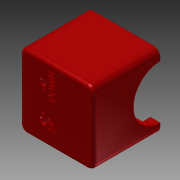
# Autodesk Inventor part: Durometer_Electronics_Enclosure_Lid
Saved by Autodesk Inventor 2015 (Build 190159000, 159)
## iProperties
Created: 2015-01-04
Part Number: Durometer_Electronics_Enclosure_Lid
Material: Generic
Document SubType Name: Modeling
Designer: Drew
Density: 1 g/cm^3
Appearance: Smooth - Red
Author: Drew
Autodesk Inventor part; units mm, degrees
ref_plane "YZ Plane" through (0, 0, 0) normal (1, 0, 0) x (0, 1, 0)
ref_plane "XZ Plane" through (0, 0, 0) normal (0, 1, 0) x (-1, 0, 0)
ref_plane "XY Plane" through (0, 0, 0) normal (0, 0, 1) x (1, 0, 0)
sketch "Sketch1" plane through (0, 0, 0) normal (0, 0, 1) x (1, 0, 0)
  line L0 (28.575, -34.925) -> (-28.575, -34.925)
  line L1 (-34.925, -28.575) -> (-34.925, 28.575)
  line L2 (-28.575, 34.925) -> (28.575, 34.925)
  line L3 (34.925, 28.575) -> (34.925, -28.575)
  line L4 (34.925, -34.925) -> (-34.925, 34.925) construction
  line L5 (-34.925, -34.925) -> (34.925, 34.925) construction
  arc A0 (-28.575, 34.925) -> (-34.925, 28.575) centre (-28.575, 28.575) ccw
  arc A1 (34.925, 28.575) -> (28.575, 34.925) centre (28.575, 28.575) ccw
  arc A2 (28.575, -34.925) -> (34.925, -28.575) centre (28.575, -28.575) ccw
  arc A3 (-34.925, -28.575) -> (-28.575, -34.925) centre (-28.575, -28.575) ccw
  point P0 (0, 0)
  dimension "d0" = 69.85
  dimension "d1" = 69.85
  dimension "d2" = 6.35
  constraints: 12 end point, 8 point on circle, 8 point on line, 8 tangent, 4 centre point, 3 equal radius, 2 midpoint, 2 parallel, 1 horizontal, 1 perpendicular
  measures "d0" distance of L4.end L5.end
  measures "d1" distance between parallel lines of L0 L2
  measures "d2" radius of A0
extrude "Extrusion1" add sketch "Sketch1" along normal blind 63.5
shell "Shell1" thickness 2.032 removed faces 1 at (9.525, 7.4083, 0)
sketch "Sketch4" plane through (0, 0, 0) normal (0, 0, -1) x (-1, 0, 0)
  arc A0 (-32.893, -28.575) -> (-28.575, -32.893) centre (-28.575, -28.575) ccw projected
  line L0 (-43.2886, 0) -> (36.2185, 0)
  line L1 (0, 45.1294) -> (0, -40.5019)
  line L2 (-28.575, -24.257) -> (-32.893, -24.257)
  line L3 (-24.257, -28.575) -> (-24.257, -32.893)
  line L4 (-24.257, -32.893) -> (-28.575, -32.893)
  line L5 (-32.893, -24.257) -> (-32.893, -28.575)
  arc A1 (-32.893, -28.575) -> (-28.575, -32.893) centre (-28.575, -28.575) ccw
  arc A2 (-24.257, -28.575) -> (-28.575, -24.257) centre (-28.575, -28.575) ccw
  arc A3 (-28.575, 32.893) -> (-32.893, 28.575) centre (-28.575, 28.575) ccw
  line L6 (-28.575, 24.257) -> (-32.893, 24.257)
  line L7 (-24.257, 28.575) -> (-24.257, 32.893)
  line L8 (-24.257, 32.893) -> (-28.575, 32.893)
  line L9 (-32.893, 24.257) -> (-32.893, 28.575)
  arc A4 (-28.575, 32.893) -> (-32.893, 28.575) centre (-28.575, 28.575) ccw
  arc A5 (-28.575, 24.257) -> (-24.257, 28.575) centre (-28.575, 28.575) ccw
  arc A6 (28.575, -32.893) -> (32.893, -28.575) centre (28.575, -28.575) ccw
  line L10 (28.575, -24.257) -> (32.893, -24.257)
  line L11 (24.257, -28.575) -> (24.257, -32.893)
  line L12 (24.257, -32.893) -> (28.575, -32.893)
  line L13 (32.893, -24.257) -> (32.893, -28.575)
  arc A7 (28.575, -32.893) -> (32.893, -28.575) centre (28.575, -28.575) ccw
  arc A8 (28.575, -24.257) -> (24.257, -28.575) centre (28.575, -28.575) ccw
  arc A9 (32.893, 28.575) -> (28.575, 32.893) centre (28.575, 28.575) ccw
  line L14 (28.575, 24.257) -> (32.893, 24.257)
  line L15 (24.257, 28.575) -> (24.257, 32.893)
  line L16 (24.257, 32.893) -> (28.575, 32.893)
  line L17 (32.893, 24.257) -> (32.893, 28.575)
  arc A10 (32.893, 28.575) -> (28.575, 32.893) centre (28.575, 28.575) ccw
  arc A11 (24.257, 28.575) -> (28.575, 24.257) centre (28.575, 28.575) ccw
  circle A12 centre (-28.575, -28.575) radius 1.45
  circle A13 centre (-28.575, 28.575) radius 1.45
  circle A14 centre (28.575, -28.575) radius 1.45
  circle A15 centre (28.575, 28.575) radius 1.45
  point P0 (0, 0)
  dimension "d7" = 4.318
  dimension "d8" = 4.318
  dimension "d11" = 2.9
  constraints: 36 end point, 27 symmetric about line, 22 point on circle, 15 centre point, 5 coincident, 4 tangent, 2 horizontal, 2 point on line, 1 vertical, 12 other
  measures "d7" distance of L2.end L5.end
  measures "d8" distance of L3.start L3.end
  measures "d11" diameter of A12
extrude "Extrusion2" add sketch "Sketch4" against normal up to surface (61.468 mm away)
fillet "Fillet2" radius 3.175 24 edges at (33.0651, 33.0651, 63.5) (0, 34.925, 63.5) (-33.0651, 33.0651, 63.5) (-34.925, 0, 63.5) (-33.0651, -33.0651, 63.5) (0, -34.925, 63.5) (33.0651, -33.0651, 63.5) (34.925, 0, 63.5) (32.893, 0, 61.468) (24.257, -30.734, 61.468) (30.734, -24.257, 61.468) (25.5217, -25.5217, 61.468) (0, -32.893, 61.468) (0, 32.893, 61.468) (30.734, 24.257, 61.468) (24.257, 30.734, 61.468) (25.5217, 25.5217, 61.468) (-30.734, -24.257, 61.468) (-24.257, -30.734, 61.468) (-25.5217, -25.5217, 61.468) (-32.893, 0, 61.468) (-24.257, 30.734, 61.468) (-30.734, 24.257, 61.468) (-25.5217, 25.5217, 61.468)
sketch "Sketch5" plane through (0, 0, 63.5) normal (0, 0, 1) x (1, 0, 0)
  circle A0 centre (-12.7, -15.875) radius 3.429
  line L0 (-50.1018, 0) -> (45.2159, 0)
  line L1 (-12.7, -24.1987) -> (-12.7, -7.4873)
  line L2 (-11.43, -9.144) -> (-13.97, -9.144)
  line L3 (-13.97, -9.144) -> (-13.97, -10.414)
  line L4 (-13.97, -10.414) -> (-11.43, -10.414)
  line L5 (-11.43, -10.414) -> (-11.43, -9.144)
  line L6 (-11.43, -9.144) -> (-13.97, -10.414) construction
  line L7 (-13.97, -9.144) -> (-11.43, -10.414) construction
  circle A1 centre (-12.7, 15.875) radius 3.429
  line L8 (-12.7, 24.1987) -> (-12.7, 7.4873)
  line L9 (-11.43, 9.144) -> (-13.97, 9.144)
  line L10 (-13.97, 9.144) -> (-13.97, 10.414)
  line L11 (-13.97, 10.414) -> (-11.43, 10.414)
  line L12 (-11.43, 10.414) -> (-11.43, 9.144)
  line L13 (-11.43, 9.144) -> (-13.97, 10.414) construction
  line L14 (-13.97, 9.144) -> (-11.43, 10.414) construction
  point P0 (0, 0)
  point P1 (-12.7, -9.779)
  point P2 (-12.7, 9.779)
  dimension "d31" = 6.096
  dimension "d32" = 6.858
  dimension "d33" = 2.54
  dimension "d34" = 1.27
  dimension "d35" = 31.75
  dimension "d36" = 12.7
  constraints: 30 end point, 8 symmetric about line, 4 midpoint, 3 point on line, 2 centre point, 2 horizontal, 2 parallel, 1 perpendicular, 1 vertical, 1 other
  measures "d31" distance of A0.centre point (-12.7, -9.779)
  measures "d32" diameter of A0
  measures "d33" distance of L2.start L2.end
  measures "d34" distance of L2.end L3.end
  measures "d35" diameter of A0.centre L0
  measures "d36" horizontal distance of point (0, 0) A0.centre
extrude "Extrusion3" cut sketch "Sketch5" against normal through all
sketch "Sketch6" plane through (0, 0, 63.5) normal (0, 0, 1) x (1, 0, 0)
  line L0 (-8.5246, -20.4603) -> (-8.5246, -15.2971) construction
  line L1 (-8.5246, -15.2971) -> (-5.3496, -15.2971) construction
  line L2 (-5.3496, -15.2971) -> (-5.3496, -20.4603) construction
  line L3 (-5.3496, -20.4603) -> (-8.5246, -20.4603) construction
  line L4 (-7.8723, 3.9052) -> (-7.8723, 16.5422) construction
  line L5 (-7.8723, 16.5422) -> (-4.6973, 16.5422) construction
  line L6 (-4.6973, 16.5422) -> (-4.6973, 3.9052) construction
  line L7 (-4.6973, 3.9052) -> (-7.8723, 3.9052) construction
  spline S0 degree 2 poles (-2.3002, -17.7136) (-2.3002, -18.2521) (-2.5818, -19.0523) (-2.8633, -19.3339) knots 0 0 0 1 2 2 2
  spline S1 degree 2 poles (-2.8633, -19.3339) (-3.1795, -19.655) (-4.0687, -19.9168) (-4.7208, -19.9168) knots 0 0 0 1 2 2 2
  line L8 (-4.7208, -19.9168) -> (-8.5246, -19.9168)
  line L9 (-8.5246, -19.9168) -> (-8.5246, -19.1067)
  line L10 (-8.5246, -19.1067) -> (-4.7208, -19.1067)
  spline S2 degree 2 poles (-4.7208, -19.1067) (-4.296, -19.1067) (-3.7229, -18.998) (-3.4907, -18.8449) knots 0 0 0 1 2 2 2
  spline S3 degree 2 poles (-3.4907, -18.8449) (-3.2437, -18.6818) (-2.9918, -18.1187) (-2.9918, -17.7136) knots 0 0 0 1 2 2 2
  spline S4 degree 2 poles (-2.9918, -17.7136) (-2.9918, -17.3332) (-3.2437, -16.7404) (-3.4907, -16.5774) knots 0 0 0 1 2 2 2
  spline S5 degree 2 poles (-3.4907, -16.5774) (-3.7229, -16.4242) (-4.291, -16.3156) (-4.701, -16.3156) knots 0 0 0 1 2 2 2
  line L11 (-4.701, -16.3156) -> (-8.5246, -16.3156)
  line L12 (-8.5246, -16.3156) -> (-8.5246, -15.5054)
  line L13 (-8.5246, -15.5054) -> (-4.7208, -15.5054)
  spline S6 degree 2 poles (-4.7208, -15.5054) (-4.0835, -15.5054) (-3.1746, -15.7623) (-2.8633, -16.0883) knots 0 0 0 1 2 2 2
  spline S7 degree 2 poles (-2.8633, -16.0883) (-2.5768, -16.3798) (-2.3002, -17.1504) (-2.3002, -17.7136) knots 0 0 0 1 2 2 2
  spline S8 degree 2 poles (-6.6869, -10.4913) (-6.2917, -10.4913) (-5.5804, -10.7728) (-5.3334, -11.0248) knots 0 0 0 1 2 2 2
  spline S9 degree 2 poles (-5.3334, -11.0248) (-5.0221, -11.341) (-4.701, -12.1956) (-4.701, -12.8477) knots 0 0 0 1 2 2 2
  line L14 (-4.701, -12.8477) -> (-4.701, -13.5343)
  line L15 (-4.701, -13.5343) -> (-2.4286, -13.5343)
  line L16 (-2.4286, -13.5343) -> (-2.4286, -14.3445)
  line L17 (-2.4286, -14.3445) -> (-8.5246, -14.3445)
  line L18 (-8.5246, -14.3445) -> (-8.5246, -12.8131)
  spline S10 degree 2 poles (-8.5246, -12.8131) (-8.5246, -12.2697) (-8.3468, -11.5089) (-8.1442, -11.2175) knots 0 0 0 1 2 2 2
  spline S11 degree 2 poles (-8.1442, -11.2175) (-7.9121, -10.8766) (-7.1957, -10.4913) (-6.6869, -10.4913) knots 0 0 0 1 2 2 2
  spline S12 degree 2 poles (-6.6622, -11.336) (-6.9784, -11.336) (-7.4428, -11.5534) (-7.591, -11.7757) knots 0 0 0 1 2 2 2
  spline S13 degree 2 poles (-7.591, -11.7757) (-7.7194, -11.9683) (-7.8231, -12.4821) (-7.8231, -12.8625) knots 0 0 0 1 2 2 2
  line L19 (-7.8231, -12.8625) -> (-7.8231, -13.5343)
  line L20 (-7.8231, -13.5343) -> (-5.3926, -13.5343)
  line L21 (-5.3926, -13.5343) -> (-5.3926, -12.981)
  spline S14 degree 2 poles (-5.3926, -12.981) (-5.3926, -12.487) (-5.5507, -11.8794) (-5.7582, -11.6818) knots 0 0 0 1 2 2 2
  spline S15 degree 2 poles (-5.7582, -11.6818) (-5.941, -11.499) (-6.3708, -11.336) (-6.6622, -11.336) knots 0 0 0 1 2 2 2
  spline S16 degree 2 poles (-4.6909, 9.3293) (-3.8561, 9.3293) (-2.5124, 8.6525) (-2.1369, 8.0844) knots 0 0 0 1 2 2 2
  spline S17 degree 2 poles (-2.1369, 8.0844) (-1.8455, 7.6201) (-1.6479, 6.6666) (-1.6479, 5.9256) knots 0 0 0 1 2 2 2
  line L22 (-1.6479, 5.9256) -> (-1.6479, 4.5227)
  line L23 (-1.6479, 4.5227) -> (-7.7439, 4.5227)
  line L24 (-7.7439, 4.5227) -> (-7.7439, 5.9108)
  spline S18 degree 2 poles (-7.7439, 5.9108) (-7.7439, 6.7704) (-7.487, 7.7485) (-7.2598, 8.0943) knots 0 0 0 1 2 2 2
  spline S19 degree 2 poles (-7.2598, 8.0943) (-6.8695, 8.6822) (-5.5802, 9.3293) (-4.6909, 9.3293) knots 0 0 0 1 2 2 2
  spline S20 degree 2 poles (-4.7008, 8.4846) (-5.4023, 8.4846) (-6.3953, 8.0202) (-6.6768, 7.5608) knots 0 0 0 1 2 2 2
  spline S21 degree 2 poles (-6.6768, 7.5608) (-6.8695, 7.2347) (-7.0424, 6.4987) (-7.0424, 5.9503) knots 0 0 0 1 2 2 2
  line L25 (-7.0424, 5.9503) -> (-7.0424, 5.3328)
  line L26 (-7.0424, 5.3328) -> (-2.3494, 5.3328)
  line L27 (-2.3494, 5.3328) -> (-2.3494, 5.9503)
  spline S22 degree 2 poles (-2.3494, 5.9503) (-2.3494, 6.4888) (-2.5223, 7.3039) (-2.7545, 7.6349) knots 0 0 0 1 2 2 2
  spline S23 degree 2 poles (-2.7545, 7.6349) (-3.041, 8.0597) (-3.9895, 8.4846) (-4.7008, 8.4846) knots 0 0 0 1 2 2 2
  spline S24 degree 2 poles (-7.0473, 14.5213) (-6.6423, 14.8671) (-5.4567, 15.2524) (-4.6959, 15.2524) knots 0 0 0 1 2 2 2
  spline S25 degree 2 poles (-4.6959, 15.2524) (-3.9549, 15.2524) (-2.7545, 14.877) (-2.3494, 14.5213) knots 0 0 0 1 2 2 2
  spline S26 degree 2 poles (-2.3494, 14.5213) (-1.9245, 14.1459) (-1.5194, 13.1529) (-1.5194, 12.5552) knots 0 0 0 1 2 2 2
  spline S27 degree 2 poles (-1.5194, 12.5552) (-1.5194, 11.9377) (-1.9393, 10.9497) (-2.3494, 10.589) knots 0 0 0 1 2 2 2
  spline S28 degree 2 poles (-2.3494, 10.589) (-2.7545, 10.2383) (-3.945, 9.8628) (-4.6959, 9.8628) knots 0 0 0 1 2 2 2
  spline S29 degree 2 poles (-4.6959, 9.8628) (-5.4616, 9.8628) (-6.6274, 10.2432) (-7.0473, 10.594) knots 0 0 0 1 2 2 2
  spline S30 degree 2 poles (-7.0473, 10.594) (-7.4524, 10.9497) (-7.8723, 11.9426) (-7.8723, 12.5552) knots 0 0 0 1 2 2 2
  spline S31 degree 2 poles (-7.8723, 12.5552) (-7.8723, 13.1776) (-7.4376, 14.1755) (-7.0473, 14.5213) knots 0 0 0 1 2 2 2
  spline S32 degree 2 poles (-4.6959, 14.4077) (-5.2986, 14.4077) (-6.2322, 14.1459) (-6.5385, 13.9087) knots 0 0 0 1 2 2 2
  spline S33 degree 2 poles (-6.5385, 13.9087) (-6.8547, 13.6667) (-7.1708, 12.9849) (-7.1708, 12.5601) knots 0 0 0 1 2 2 2
  spline S34 degree 2 poles (-7.1708, 12.5601) (-7.1708, 12.1204) (-6.8646, 11.4585) (-6.5385, 11.2065) knots 0 0 0 1 2 2 2
  spline S35 degree 2 poles (-6.5385, 11.2065) (-6.2273, 10.9645) (-5.2887, 10.7076) (-4.6959, 10.7076) knots 0 0 0 1 2 2 2
  spline S36 degree 2 poles (-4.6959, 10.7076) (-3.4955, 10.7076) (-2.2209, 11.7154) (-2.2209, 12.5601) knots 0 0 0 1 2 2 2
  spline S37 degree 2 poles (-2.2209, 12.5601) (-2.2209, 13.4048) (-3.4955, 14.4077) (-4.6959, 14.4077) knots 0 0 0 1 2 2 2
  line L28 (-7.7439, 22.9737) -> (-1.6479, 21.4423)
  line L29 (-1.6479, 21.4423) -> (-1.6479, 20.5333)
  line L30 (-1.6479, 20.5333) -> (-6.7065, 19.2934)
  line L31 (-6.7065, 19.2934) -> (-1.6479, 18.088)
  line L32 (-1.6479, 18.088) -> (-1.6479, 17.1889)
  line L33 (-1.6479, 17.1889) -> (-7.7439, 15.6328)
  line L34 (-7.7439, 15.6328) -> (-7.7439, 16.4677)
  line L35 (-7.7439, 16.4677) -> (-2.6902, 17.6928)
  line L36 (-2.6902, 17.6928) -> (-7.7439, 18.908)
  line L37 (-7.7439, 18.908) -> (-7.7439, 19.733)
  line L38 (-7.7439, 19.733) -> (-2.631, 20.9582)
  line L39 (-2.631, 20.9582) -> (-7.7439, 22.1783)
  line L40 (-7.7439, 22.1783) -> (-7.7439, 22.9737)
  line L41 (-1.6479, 28.0619) -> (-1.6479, 27.153)
  line L42 (-1.6479, 27.153) -> (-6.9041, 24.4557)
  line L43 (-6.9041, 24.4557) -> (-1.6479, 24.4557)
  line L44 (-1.6479, 24.4557) -> (-1.6479, 23.6999)
  line L45 (-1.6479, 23.6999) -> (-7.7439, 23.6999)
  line L46 (-7.7439, 23.6999) -> (-7.7439, 24.8509)
  line L47 (-7.7439, 24.8509) -> (-2.9175, 27.3061)
  line L48 (-2.9175, 27.3061) -> (-7.7439, 27.3061)
  line L49 (-7.7439, 27.3061) -> (-7.7439, 28.0619)
  line L50 (-7.7439, 28.0619) -> (-1.6479, 28.0619)
  point P0 (0, 0)
  point P1 (-7.8723, 10.2237)
  point P2 (-8.5246, -17.8787)
  dimension "d39" = 3.175
  dimension "d40" = 3.175
  dimension "d41" = 5.1631
  dimension "d42" = 12.637
  constraints: 2 midpoint, 4 other
  measures "d39" distance of L2.end L0.start
  measures "d40" distance of L6.end L4.start
  measures "d41" distance of L1.end L2.end
  measures "d42" distance of L5.end L6.end
extrude "Extrusion4" cut sketch "Sketch6" against normal blind 1.27
sketch "Sketch7" plane through (34.925, -28.575, 0) normal (1, 0, 0) x (0, 0, -1)
  line L0 (-78.8961, 28.575) -> (28.5561, 28.575)
  arc A0 (0, 53.975) -> (0, 3.175) centre (0, 28.575) ccw
  line L1 (0, 3.175) -> (0, 53.975)
  line L2 (0, 4.318) -> (0, 52.832) projected
  point P0 (0, 28.575)
  dimension "d45" = 25.4
  constraints: 4 end point, 3 point on line, 2 point on circle, 1 centre point, 1 coincident, 1 horizontal, 1 midpoint
  measures "d45" radius of A0
extrude "Extrusion5" cut sketch "Sketch7" against normal up to next
equation "\"d1\" = d0"
equation "\"d8\" = d7"
equation "\"d40\" = d39"
body "Solid1"
